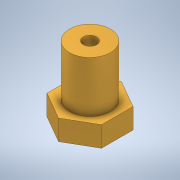
# Autodesk Inventor part: boquilla 0.4
Saved by Autodesk Inventor 2022 (Build 260153000, 153)
## iProperties
Created: 2021-10-27
Part Number: boquilla 0.4
Material: Latón, amarillo claro
Document SubType Name: Modeling
Designer: arman
Density: 8.47 g/cm^3
Appearance: Latón - Satinado
Author: arman
Autodesk Inventor part; units mm, degrees
ref_plane "YZ Plane" through (0, 0, 0) normal (1, 0, 0) x (0, 1, 0)
ref_plane "Plano de trabajo1" through (0, 8, 0) normal (0, 1, 0) x (-1, 0, 0)
sketch "Boceto2" plane through (0, 8, 0) normal (0, 1, 0) x (-1, 0, 0)
  line L0 (0, -4.6188) -> (-4, -2.3094)
  line L1 (-4, -2.3094) -> (-4, 2.3094)
  line L2 (-4, 2.3094) -> (0, 4.6188)
  line L3 (0, 4.6188) -> (4, 2.3094)
  line L4 (4, 2.3094) -> (4, -2.3094)
  line L5 (4, -2.3094) -> (0, -4.6188)
  point P0 (0, 0)
  point P1 (0, 0)
  dimension "d2" = 8
  constraints: 12 end point, 1 coincident, 13 other
  measures "d2" distance between parallel lines of L1 L4
extrude "Extrusión1" add sketch "Boceto2" against normal blind 3
sketch "Boceto3" plane through (0, 8, 0) normal (0, 1, 0) x (1, 0, 0)
  circle A0 centre (0, 0) radius 3
  circle A1 centre (0, 0) radius 3
  dimension "d9" = 6
  dimension "d10" = 6
  constraints: 2 centre point, 2 coincident
  measures "d9" diameter of A0
  measures "d10" diameter of A1
extrude "Extrusión2" add sketch "Boceto3" along normal blind 1
sketch "Boceto4" plane through (0, 9, 0) normal (0, 1, 0) x (1, 0, 0)
  circle A0 centre (0, 0) radius 3 projected
extrude "Extrusión3" add sketch "Boceto4" along normal blind 6.5
sketch "Boceto6" plane through (0, 15.5, 0) normal (0, 1, 0) x (1, 0, 0)
  circle A0 centre (0, 0) radius 1
  dimension "d26" = 2
  constraints: 1 centre point
  measures "d26" diameter of A0
extrude "Extrusión4" cut sketch "Boceto6" against normal blind 12.25
sketch "Boceto12" plane through (0, 5, 0) normal (0, -1, 0) x (1, 0, 0)
  circle A0 centre (0, 0) radius 1
  line L0 (-1.8028, 3) -> (1.8028, 3)
  arc A1 (1.8028, -3) -> (1.8028, 3) centre (0, 0) ccw
  arc A2 (-1.8028, 3) -> (-1.8028, -3) centre (0, 0) ccw
  line L1 (1.8028, -3) -> (-1.8028, -3)
  constraints: 4 end point, 4 point on circle, 3 centre point, 2 horizontal, 1 coincident
ref_plane "Plano de trabajo6" through (0, 3.8, 0) normal (0, -1, 0) x (1, 0, 0)
ref_plane "Plano de trabajo5" through (0, 3, 0) normal (0, -1, 0) x (1, 0, 0)
sketch "Boceto13" plane through (0, 3, 0) normal (0, -1, 0) x (1, 0, 0)
  circle A0 centre (0, 0) radius 0.2
  dimension "d44" = 0.4
  constraints: 1 centre point, 1 coincident
  measures "d44" diameter of A0
sketch "Boceto14" plane through (0, 3.8, 0) normal (0, -1, 0) x (1, 0, 0)
  circle A0 centre (0, 0) radius 0.2
  dimension "d45" = 0.4
  constraints: 1 centre point, 1 coincident
  measures "d45" diameter of A0
loft "Solevación2" add profiles "Boceto12", "Boceto13" contours A0 | L0 A1 L1 A2 / all
loft "Solevación3" cut profiles "Boceto14" section 2 edges at (-1, 5, 0)
sketch "Boceto15" plane through (0, 3, 0) normal (0, -1, 0) x (0.9991294, 0, 0.0417196)
  circle A0 centre (0, 0) radius 0.2
  dimension "d54" = 0.4
  constraints: 1 centre point, 1 coincident
  measures "d54" diameter of A0
extrude "Extrusión8" cut sketch "Boceto15" against normal blind 2
